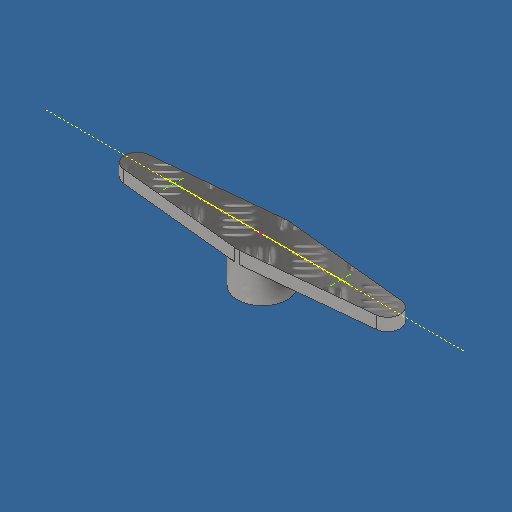
# Autodesk Inventor part: motor_adaptator
Saved by Autodesk Inventor 2025 (Build 290162000, 162)
## iProperties
Created: 2024-11-29
Part Number: motor_adaptator
Material: Generic
Document SubType Name: Modeling
Designer: Pauline Simonnet
Density: 1 g/cm^3
Appearance: Diamond Plate
Author: Pauline Simonnet
Autodesk Inventor part; units mm, degrees
ref_plane "YZ Plane" through (0, 0, 0) normal (1, 0, 0) x (0, 1, 0)
ref_plane "XZ Plane" through (0, 0, 0) normal (0, 1, 0) x (-1, 0, 0)
ref_plane "XY Plane" through (0, 0, 0) normal (0, 0, 1) x (1, 0, 0)
sketch "Sketch1" plane through (0, 0, 0) normal (0, 1, 0) x (-1, 0, 0)
  circle A0 centre (0, 0) radius 2.5
  circle A1 centre (0, 0) radius 4
  dimension "d0" = 5
  dimension "d1" = 1.5
  constraints: 2 centre point, 2 coincident
  measures "d0" diameter of A0
  measures "d1" radial gap between concentric circles of A1 A0
extrude "Extrusion1" add sketch "Sketch1" along normal blind 5
sketch "Sketch2" plane through (0, 5, 0) normal (0, 1, 0) x (1, 0, 0)
  circle A0 centre (0, 0) radius 4 projected
  circle A1 centre (-20, 0) radius 2
  line L0 (-20.2, -1.99) -> (-0.4, -3.9799)
  line L1 (-20.2, 1.99) -> (-0.4, 3.9799)
  line L2 (0, -12.1879) -> (0, 12.2069) construction
  circle A2 centre (20, 0) radius 2
  line L3 (20.2, -1.99) -> (0.4, -3.9799)
  line L4 (20.2, 1.99) -> (0.4, 3.9799)
  circle A3 centre (0, 0) radius 4 construction
  dimension "d15" = 4
  dimension "d16" = 0
  dimension "d17" = 20
  constraints: 10 end point, 6 point on circle, 5 symmetric about line, 5 tangent, 2 centre point, 1 vertical, 1 other
  measures "d15" diameter of A1
  measures "d16" vertical distance of point (0, 0) A1.centre
  measures "d17" distance of point (0, 0) A1.centre
extrude "Extrusion2" add sketch "Sketch2" along normal blind 2
sketch "Sketch3" plane through (0, 7, 0) normal (0, 1, 0) x (1, 0, 0)
  line L0 (32.4593, 0) -> (-34.4987, 0) construction
  point P0 (0, 0)
  point P1 (12.4993, 0)
  point P2 (-14.1195, 0)
  constraints: 2 end point, 2 point on line, 1 horizontal
sketch "Sketch4" plane through (0, 5, 0) normal (0, -1, 0) x (1, 0, 0)
  point P0 (0, 0)
  point P1 (0, 0)
  constraints: 1 coincident
ref_plane "Work Plane1" through (-14.1195, 7, 0) normal (0, 0, -1) x (1, 0, 0)
body "Solid1"
